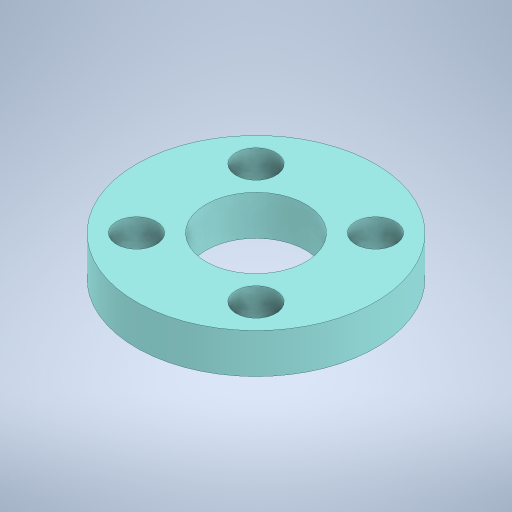
# Autodesk Inventor part: Flip up and down (shaft to motor ring)
Saved by Autodesk Inventor 2023.1 (Build 271208000, 208)
## iProperties
Created: 2022-12-20
Part Number: Flip up and down (shaft to motor ring)
Material: Generic
Document SubType Name: Modeling
Designer: shubh
Density: 1 g/cm^3
Appearance: Default(2)
Author: shubh
Autodesk Inventor part; units mm, degrees
ref_plane "YZ Plane" through (0, 0, 0) normal (1, 0, 0) x (0, 1, 0)
ref_plane "XZ Plane" through (0, 0, 0) normal (0, 1, 0) x (-1, 0, 0)
ref_plane "XY Plane" through (0, 0, 0) normal (0, 0, 1) x (1, 0, 0)
sketch "Sketch1" plane through (0, 0, 0) normal (0, 1, 0) x (-1, 0, 0)
  circle A0 centre (0, 0) radius 9.525
  circle A1 centre (0, 0) radius 3.9751
  circle A2 centre (4.7625, 4.7625) radius 1.5875
  circle A3 centre (-4.7625, 4.7625) radius 1.5875
  circle A4 centre (-4.7625, -4.7625) radius 1.5875
  circle A5 centre (4.7625, -4.7625) radius 1.5875
  dimension "d0" = 19.05
  dimension "d1" = 7.9502
  dimension "d2" = 3.175
  dimension "d5" = 360
  constraints: 6 centre point, 2 coincident, 9 other
  measures "d0" diameter of A0
  measures "d1" diameter of A1
  measures "d2" diameter of A2
extrude "Extrusion1" add sketch "Sketch1" along normal blind 3.175
body "Solid1"
